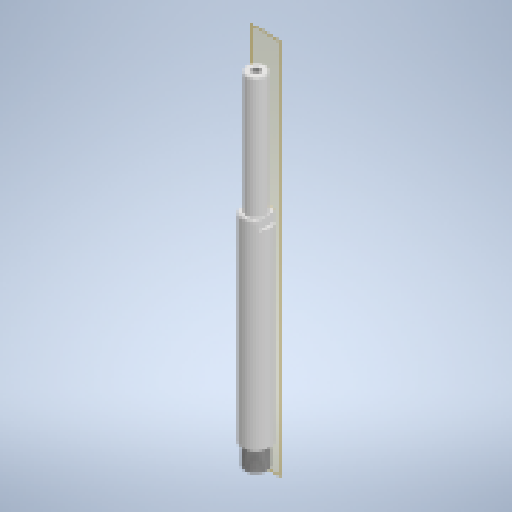
# Autodesk Inventor part: Вал
Saved by Autodesk Inventor 2023.2 (Build 272271030, 271C)
## iProperties
Created: 2024-02-27
Part Number: Вал
Material: Типовые
Document SubType Name: Modeling
Designer: user
Density: 1 g/cm^3
Appearance: По умолчанию
Author: user
Autodesk Inventor part; units mm, degrees
ref_plane "YZ Plane" through (0, 0, 0) normal (1, 0, 0) x (0, 1, 0)
ref_plane "XZ Plane" through (0, 0, 0) normal (0, 1, 0) x (-1, 0, 0)
sketch "Эскиз1" plane through (0, 0, 0) normal (0, 0, 1) x (1, 0, 0)
  line L0 (0, 137) -> (0, -200)
  line L1 (0, 137) -> (9, 137)
  line L2 (9, 137) -> (9, 25)
  line L3 (9, 25) -> (12.5, 25)
  line L4 (12.5, 25) -> (12.5, -180)
  line L5 (12.5, -180) -> (0, -180)
  line L6 (10, -180) -> (10, -160)
  line L7 (10, -160) -> (12.5, -160)
  point P0 (0, 0)
  point P1 (0, -177.0364)
  dimension "d1" = 200
  dimension "d2" = 18
  dimension "d3" = 25
  dimension "d7" = 25
  dimension "d8" = 137
  dimension "d16" = 180
  dimension "d17" = 20
  dimension "d18" = 20
  constraints: 16 end point, 5 perpendicular, 5 point on line, 2 horizontal, 1 vertical
  measures "d1" distance of point (0, 0) L0.end
  measures "d2" diameter of L2 L0
  measures "d3" diameter of L4 L0
  measures "d7" distance from line of point (0, 0) L3
  measures "d8" distance from line of point (0, 0) L1
  measures "d16" distance from line of point (0, 0) L5
  measures "d17" diameter of L6 L0
  measures "d18" distance of L6.start L6.end
revolve "Вращение1" add sketch "Эскиз1" angle 360 about axis through (0, 137, 0) along (0, -1, 0) contours L1 L2 L3 L4 L7 L6 L5 L0
sketch "Эскиз2" plane through (0, 137, 0) normal (0, 1, 0) x (1, 0, 0)
  point P0 (0, 0)
hole "Отверстие1" at (0, 137, 0) direction (0, -1, 0) diameter 6.647 depth 30 tip angle 118 thread size "M8x1.25" class "6H" standard "ISO Metric profile"
thread "Резьба1" size "M20x2.5" class "6g" standard "ISO Metric profile" full length
ref_plane "РабПлоскость1" through (0, 81, -9) normal (0, 0, 1) x (1, 0, 0)
sketch "Эскиз3" plane through (0, 81, -9) normal (0, 0, 1) x (1, 0, 0)
  line L0 (0, 46) -> (0, -24) construction
  line L1 (-2.55, 46) -> (-2.55, -24)
  line L2 (2.55, -24) -> (2.55, 46)
  arc A0 (2.55, 46) -> (-2.55, 46) centre (0, 46) ccw
  arc A1 (-2.55, -24) -> (2.55, -24) centre (0, -24) ccw
  line L3 (-9, 56) -> (9, 56) projected
  point P0 (0, -81)
  point P1 (0, 11)
  point P2 (0, 56)
  dimension "d21" = 10
  dimension "d22" = 70
  dimension "d23" = 5.1
  constraints: 8 end point, 4 point on circle, 4 tangent, 2 centre point, 2 midpoint, 1 parallel, 1 vertical, 1 vertical alignment
  measures "d21" distance from line of L0.start L3
  measures "d22" distance of L0.start L0.end
  measures "d23" distance between parallel lines of L1 L2
extrude "Выдавливание1" cut sketch "Эскиз3" along normal blind 2
chamfer "Chamfer1" distance 1 angle 45 4 edges at (-9, 137, 0) (-12.5, 25, 0) (-12.5, -160, 0) (-10, -180, 0)
sketch "Sketch4" plane through (0, 0, 0) normal (0, 0, 1) x (1, 0, 0)
  line L0 (12.5, 24) -> (-12.5, 24) projected
  line L1 (-12.5, -159) -> (12.5, -159) projected
  line L2 (-11.5, 25) -> (11.5, 25) projected
  line L3 (12.5, 24) -> (-12.5, 24) projected
  line L4 (-11.5, 25) -> (11.5, 25) projected
  line L5 (9.5, 25) -> (9.5, 17)
  line L6 (9.5, 17) -> (12.5, 17)
  line L7 (-12.5, 17) -> (-9.5, 17)
  line L8 (-9.5, 17) -> (-9.5, 25)
  line L9 (-9, 25) -> (9, 25) projected
  line L10 (0, 25) -> (0, 9.8425) construction
  line L11 (12.5, 24) -> (-12.5, 24) projected
  line L12 (12.5, 24) -> (12.5, 17)
  line L13 (11.5, 25) -> (12.5, 24)
  line L14 (11.5, 25) -> (12.5, 24) projected
  line L15 (-11.5, 25) -> (-12.5, 24)
  line L16 (-11.5, 25) -> (-12.5, 24) projected
  line L17 (-12.5, 17) -> (-12.5, 24)
  line L18 (-12.5, 24) -> (-12.5, -159) projected
  point P0 (0, 0)
  dimension "d29" = 19
  dimension "d30" = 8
  constraints: 18 end point, 4 perpendicular, 3 collinear, 2 point on line, 1 horizontal, 1 midpoint, 1 vertical, 2 other
  measures "d29" distance between parallel lines of L8 L5
  measures "d30" distance of L5.start L5.end
extrude "Extrusion2" cut sketch "Sketch4" along normal through all both and the other way through all contours L12 L6 L5 L0 | L0 L5 L2 L13 | L8 L7 L17 L0 | L0 L15 L2 L8
